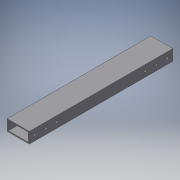
# Autodesk Inventor part: ATACHMENT BAR
Saved by Autodesk Inventor 2018 (Build 220112000, 112)
## iProperties
Created: 2019-01-26
Part Number: ATACHMENT BAR
Material: Generic
Document SubType Name: Modeling
Designer: s-4008082
Density: 1 g/cm^3
Appearance: Default
Author: s-4008082
Autodesk Inventor part; units mm, degrees
ref_plane "YZ Plane" through (0, 0, 0) normal (1, 0, 0) x (0, 1, 0)
ref_plane "XZ Plane" through (0, 0, 0) normal (0, 1, 0) x (-1, 0, 0)
ref_plane "XY Plane" through (0, 0, 0) normal (0, 0, 1) x (1, 0, 0)
sketch "Sketch1" plane through (0, 0, 0) normal (0, 0, 1) x (1, 0, 0)
  line L0 (0, 0) -> (-50.8, 0)
  line L1 (-50.8, 0) -> (-50.8, 25.4)
  line L2 (-50.8, 25.4) -> (0, 25.4)
  line L3 (0, 25.4) -> (0, 0)
  line L4 (-48.26, 22.86) -> (-2.54, 22.86)
  line L5 (-2.54, 22.86) -> (-2.54, 2.54)
  line L6 (-2.54, 2.54) -> (-48.26, 2.54)
  line L7 (-48.26, 2.54) -> (-48.26, 22.86)
  dimension "d0" = 25.4
  dimension "d1" = 50.8
  dimension "d2" = 2.54
  dimension "d3" = 2.54
  dimension "d4" = 2.54
  dimension "d5" = 2.54
  constraints: 16 end point, 4 parallel, 2 horizontal, 2 perpendicular
  measures "d0" distance of L0.end L1.end
  measures "d1" distance of L1.end L2.end
  measures "d2" distance between parallel lines of L1 L7
  measures "d3" distance between parallel lines of L2 L4
  measures "d4" distance between parallel lines of L3 L5
  measures "d5" distance between parallel lines of L0 L6
extrude "Extrusion1" add sketch "Sketch1" along normal blind 330.2
sketch "Sketch2" plane through (-50.8, 0, 0) normal (-1, 0, 0) x (0, 0, 1)
  circle A0 centre (12.7, 12.7) radius 2.5797
  circle A1 centre (38.1, 12.7) radius 2.5797
  circle A2 centre (63.5, 12.7) radius 2.5797
  circle A3 centre (266.7, 12.7) radius 2.5797
  circle A4 centre (292.1, 12.7) radius 2.5797
  circle A5 centre (317.5, 12.7) radius 2.5797
  line L0 (0, 0) -> (0, 25.4) projected
  line L1 (330.2, 25.4) -> (330.2, 0) projected
  line L2 (0, 25.4) -> (330.2, 25.4) projected
  dimension "d8" = 12.7
  dimension "d9" = 25.4
  dimension "d10" = 25.4
  dimension "d11" = 25.4
  dimension "d12" = 25.4
  dimension "d13" = 12.7
  dimension "d14" = 5.1594
  dimension "d15" = 5.1594
  dimension "d16" = 5.1594
  dimension "d19" = 5.1594
  dimension "d20" = 5.1594
  dimension "d21" = 5.1594
  dimension "d22" = 12.7
  dimension "d23" = 12.7
  dimension "d24" = 12.7
  dimension "d25" = 12.7
  dimension "d26" = 12.7
  dimension "d27" = 12.7
  constraints: 6 centre point
  measures "d8" distance from line of L0 A0.centre
  measures "d9" distance of A0.centre A1.centre
  measures "d10" distance of A1.centre A2.centre
  measures "d11" distance of A4.centre A3.centre
  measures "d12" distance of A4.centre A5.centre
  measures "d13" distance from line of L1 A5.centre
  measures "d14" diameter of A5
  measures "d15" diameter of A4
  measures "d16" diameter of A3
  measures "d19" diameter of A2
  measures "d20" diameter of A1
  measures "d21" diameter of A0
  measures "d22" distance from line of L2 A2.centre
  measures "d23" distance from line of L2 A1.centre
  measures "d24" distance from line of L2 A0.centre
  measures "d25" distance from line of L2 A3.centre
  measures "d26" distance from line of L2 A4.centre
  measures "d27" distance from line of L2 A5.centre
extrude "Extrusion2" cut sketch "Sketch2" against normal blind 279.4
sketch "Sketch3" plane through (-50.8, 0, 0) normal (0, -1, 0) x (1, 0, 0)
  circle A0 centre (12.7, 293.8134) radius 2.5797
  circle A1 centre (38.1, 293.8134) radius 2.5797
  line L0 (0, 0) -> (0, 330.2) projected
  point P0 (50.8, 0)
  dimension "d30" = 5.1594
  dimension "d31" = 5.1594
  dimension "d32" = 12.7
  dimension "d33" = 25.4
  constraints: 2 centre point
  measures "d30" diameter of A1
  measures "d31" diameter of A0
  measures "d32" distance from line of L0 A0.centre
  measures "d33" distance of A0.centre A1.centre
extrude "Extrusion3" cut sketch "Sketch3" against normal blind 279.4
equation "\"d10\" = d9"
equation "\"d11\" = d9"
equation "\"d15\" = d14"
equation "\"d16\" = d14"
equation "\"d19\" = d14"
equation "\"d20\" = d14"
equation "\"d21\" = d14"
equation "\"d26\" = d25"
equation "\"d27\" = d25"
equation "\"d31\" = d30"
body "Solid1"
